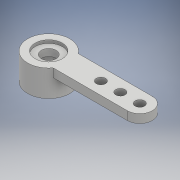
# Autodesk Inventor part: hone
Saved by Autodesk Inventor 2017 (Build 210142000, 142)
## iProperties
Part Number: hone
Material: 一般
Document SubType Name: Modeling
Designer: sktom
Density: 1 g/cm^3
Appearance: 既定
Author: sktom
Autodesk Inventor part; units mm, degrees
ref_plane "YZ Plane" through (0, 0, 0) normal (1, 0, 0) x (0, 1, 0)
ref_plane "XZ Plane" through (0, 0, 0) normal (0, 1, 0) x (-1, 0, 0)
ref_plane "XY Plane" through (0, 0, 0) normal (0, 0, 1) x (1, 0, 0)
sketch "スケッチ1" plane through (0, 0, 0) normal (0, 0, 1) x (1, 0, 0)
  circle A0 centre (0, 0) radius 2.7
  circle A1 centre (0, 0) radius 0.95
  dimension "d0" = 5.4
  dimension "d1" = 1.9
  constraints: 2 centre point, 2 coincident
  measures "d0" diameter of A0
  measures "d1" diameter of A1
extrude "押し出し1" add sketch "スケッチ1" along normal blind 3.4
sketch "スケッチ2" plane through (0, 0, 3.4) normal (0, 0, 1) x (1, 0, 0)
  circle A0 centre (0, 0) radius 1.75
  dimension "d4" = 3.5
  constraints: 1 centre point, 1 coincident
  measures "d4" diameter of A0
extrude "押し出し2" cut sketch "スケッチ2" against normal blind 0.4
sketch "スケッチ3" plane through (0, 0, 0) normal (0, 0, -1) x (-1, 0, 0)
  circle A0 centre (0, 0) radius 0.95 projected
  circle A1 centre (0, 0) radius 1.9
  dimension "d7" = 3.8
  constraints: 1 centre point, 1 coincident
  measures "d7" diameter of A1
extrude "押し出し3" cut sketch "スケッチ3" against normal blind 2.1
sketch "スケッチ4" plane through (0, 0, 3.4) normal (0, 0, 1) x (1, 0, 0)
  arc A0 (11.7, -1.6) -> (11.7, 1.6) centre (11.7, 0) ccw
  line L0 (11.7, 1.6) -> (2.1749, 1.6)
  circle A1 centre (0, 0) radius 2.7 projected
  line L1 (11.7, -1.6) -> (2.1749, -1.6)
  circle A2 centre (0, 0) radius 2.7 projected
  arc A3 (2.1749, -1.6) -> (2.1749, 1.6) centre (0, 0) ccw
  dimension "d10" = 11.7
  dimension "d11" = 3.2
  constraints: 4 end point, 4 point on circle, 2 centre point, 2 tangent, 1 coincident, 1 horizontal, 1 horizontal alignment, 1 parallel, 4 other
  measures "d10" distance of point (0, 0) A0.centre
  measures "d11" diameter of A0
extrude "押し出し4" add sketch "スケッチ4" against normal blind 1.1 contours L1 A1 L0 A0
sketch "スケッチ5" plane through (0, 0, 3.4) normal (0, 0, 1) x (1, 0, 0)
  arc A0 (11.7, -1.6) -> (11.7, 1.6) centre (11.7, 0) ccw projected
  circle A1 centre (11.7, 0) radius 0.6
  circle A2 centre (9.2, 0) radius 0.6
  circle A3 centre (6.7, 0) radius 0.6
  point P0 (0, 0)
  dimension "d14" = 1.2
  dimension "d15" = 2.5
  dimension "d16" = 2.5
  constraints: 3 centre point, 2 equal radius, 2 horizontal alignment, 1 coincident
  measures "d14" diameter of A1
  measures "d15" distance of A2.centre A1.centre
  measures "d16" distance of A3.centre A2.centre
extrude "押し出し5" cut sketch "スケッチ5" against normal up to next
